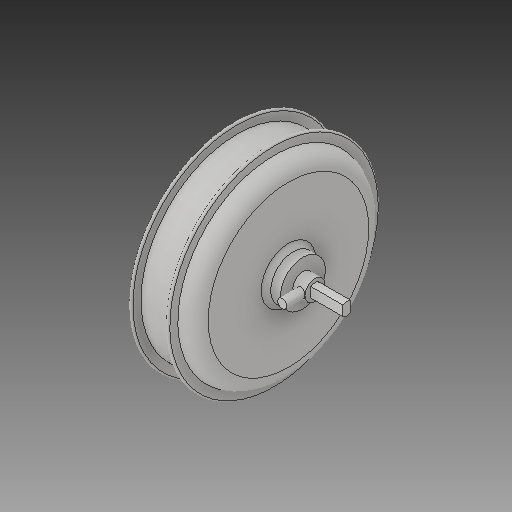
# Autodesk Inventor part: HubMotor3KW
Saved by Autodesk Inventor 2019.2 (Build 232265000, 265)
## iProperties
Created: 2018-06-05
Part Number: HubMotor3KW
Material: Generic
Document SubType Name: Modeling
Designer: eroldan
Density: 1 g/cm^3
Appearance: Default
Author: eroldan
Autodesk Inventor part; units mm, degrees
ref_plane "YZ Plane" through (0, 0, 0) normal (1, 0, 0) x (0, 1, 0)
ref_plane "XZ Plane" through (0, 0, 0) normal (0, 1, 0) x (-1, 0, 0)
ref_plane "XY Plane" through (0, 0, 0) normal (0, 0, 1) x (1, 0, 0)
sketch "Sketch1" plane through (0, 0, 0) normal (0, 0, 1) x (1, 0, 0)
  line L0 (0, 0) -> (0, 8)
  line L1 (0, 8) -> (40, 8)
  line L2 (40, 8) -> (40, 8.5)
  line L3 (40, 8.5) -> (63.75, 8.5)
  line L4 (63.75, 8.5) -> (63.75, 22.5)
  line L5 (63.75, 22.5) -> (78, 22.5)
  line L6 (78, 22.5) -> (78, 120)
  line L7 (78, 120) -> (86, 120)
  line L8 (86, 120) -> (86, 132)
  line L9 (86, 132) -> (90, 132)
  line L10 (90, 132) -> (90, 120)
  line L11 (90, 120) -> (132, 120)
  line L12 (132, 120) -> (132, 132)
  line L13 (132, 132) -> (136, 132)
  line L14 (136, 132) -> (136, 120)
  line L15 (136, 120) -> (154, 120)
  line L16 (154, 120) -> (154, 28)
  line L17 (154, 28) -> (172, 28)
  line L18 (172, 28) -> (172, 12.5)
  line L19 (172, 12.5) -> (187, 12.5)
  line L20 (187, 12.5) -> (187, 8)
  line L21 (187, 8) -> (227, 8)
  line L22 (227, 8) -> (227, 0)
  line L23 (0, 0) -> (227, 0)
  line L24 (-45.4, 0) -> (272.4, 0) projected
  point P0 (111, 120)
  point P1 (32, 8)
  dimension "d0" = 8
  dimension "d1" = 8
  dimension "d2" = 46
  dimension "d3" = 8.5
  dimension "d4" = 14.25
  dimension "d5" = 23.75
  dimension "d6" = 22.5
  dimension "d7" = 40
  dimension "d8" = 4
  dimension "d9" = 12
  dimension "d11" = 4
  dimension "d12" = 50
  dimension "d14" = 28
  dimension "d16" = 36
  dimension "d18" = 15
  dimension "d19" = 12.5
  dimension "d20" = 40
  dimension "d21" = 18
  dimension "d22" = 147
  dimension "d38" = 120
  dimension "d52" = 76
  dimension "d54" = 8
  dimension "d55" = 79
  dimension "d56" = 155
  constraints: 48 end point, 17 perpendicular, 4 horizontal alignment, 3 horizontal, 3 point on line, 3 vertical, 1 midpoint
  measures "d0" distance of L0.start L0.end
  measures "d1" distance of L6.end L7.end
  measures "d2" horizontal distance of L2.end L8.end
  measures "d3" distance from line of L0.start L3
  measures "d4" distance of L4.end L5.end
  measures "d5" distance of L2.end L3.end
  measures "d6" vertical distance of L0.start L5.end
  measures "d7" distance of L0.end L1.end
  measures "d8" distance of L8.end L9.end
  measures "d9" distance of L9.end L10.end
  measures "d11" distance of L12.end L13.end
  measures "d12" distance between parallel lines of L14 L8
  measures "d14" vertical distance of L16.end L22.end
  measures "d16" horizontal distance of L17.end L14.end
  measures "d18" distance of L18.end L19.end
  measures "d19" vertical distance of L22.end L19.end
  measures "d20" distance of L20.end L21.end
  measures "d21" distance of L14.end L15.end
  measures "d22" distance between parallel lines of L2 L20
  measures "d38" distance between parallel lines of L24 L11
  measures "d52" distance from line of L20 point (111, 120)
  measures "d54" distance of point (32, 8) L1.end
  measures "d55" horizontal distance of point (32, 8) point (111, 120)
  measures "d56" distance of point (32, 8) L20.end
revolve "Revolution1" add sketch "Sketch1" angle 360 about axis through (-10, 0, 0) along (1, 0, 0)
fillet "Fillet1" radius 20 1 edges at (154, -120, 0)
fillet "Fillet2" radius 6 1 edges at (78, -120, 0)
fillet "Fillet4" radius 2 4 edges at (132, -132, 0) (136, -132, 0) (86, -132, 0) (90, -132, 0)
fillet "Fillet6" radius 6 1 edges at (154, -28, 0)
sketch "Sketch2" plane through (0, 0, 0) normal (-1, 0, 0) x (0, 0, 1)
  line L0 (5, -10) -> (-5, -10)
  line L1 (-5, -10) -> (-5, 10)
  line L2 (-5, 10) -> (5, 10)
  line L3 (5, 10) -> (5, -10)
  line L4 (5, -10) -> (-5, 10) construction
  line L5 (-5, -10) -> (5, 10) construction
  line L6 (-13, 18) -> (-13, -18)
  line L7 (-13, -18) -> (13, -18)
  line L8 (13, -18) -> (13, 18)
  line L9 (13, 18) -> (-13, 18)
  point P0 (0, 0)
  dimension "d29" = 10
  dimension "d30" = 20
  dimension "d31" = 8
  constraints: 20 end point, 4 parallel, 2 midpoint, 2 perpendicular, 1 horizontal, 3 other
  measures "d29" distance of L1.end L2.end
  measures "d30" distance of L0.end L1.end
  measures "d31" distance from line of L2.end L8
extrude "Extrusion1" cut sketch "Sketch2" against normal up to surface (40 mm away)
sketch "Sketch3" plane through (227, 0, 0) normal (1, 0, 0) x (0, 0, -1)
  line L0 (-13, 18) -> (13, 18) projected
  line L1 (13, 18) -> (13, -18) projected
  line L2 (13, -18) -> (-13, -18) projected
  line L3 (5, 10) -> (-5, 10) projected
  line L4 (5, -10) -> (5, 10) projected
  line L5 (-5, -10) -> (5, -10) projected
  line L6 (-5, 10) -> (-5, -10) projected
  line L7 (-13, -18) -> (-13, 18) projected
  point P0 (0, 0)
extrude "Extrusion2" cut sketch "Sketch3" against normal up to surface (40 mm away)
sketch "Sketch6" plane through (40, 0, 0) normal (-1, 0, 0) x (0, 0, 1)
  circle A0 centre (0, 0) radius 12.5 projected
  arc A1 (5, 6.245) -> (-5, 6.245) centre (0, 0) ccw projected
  line L0 (-5, -6.245) -> (-5, 6.245) projected
  arc A2 (-5, -6.245) -> (5, -6.245) centre (0, 0) ccw projected
  line L1 (5, 6.245) -> (5, -6.245) projected
  arc A3 (5.7, 6.5727) -> (-5.7, 6.5727) centre (0, 0) ccw
  line L2 (5.7, 6.5727) -> (5.7, -6.5727)
  arc A4 (-5.7, -6.5727) -> (5.7, -6.5727) centre (0, 0) ccw
  line L3 (-5.7, -6.5727) -> (-5.7, 6.5727)
  dimension "d44" = 0.7
  constraints: 4 end point, 4 point on circle, 2 centre point, 3 other
  measures "d44" radial gap between concentric circles of A1 A3
extrude "Extrusion5" add sketch "Sketch6" along normal blind 4 separate body contours A0
sketch "Sketch7" plane through (36, 0, 0) normal (-1, 0, 0) x (0, 0, 1)
  line L0 (5.7, 6.5727) -> (5.7, -6.5727) projected
  arc A0 (-5.7, -6.5727) -> (5.7, -6.5727) centre (0, 0) ccw projected
  line L1 (-5.7, -6.5727) -> (-5.7, 6.5727) projected
  arc A1 (5.7, 6.5727) -> (-5.7, 6.5727) centre (0, 0) ccw projected
  circle A2 centre (0, 0) radius 12.5 projected
extrude "Extrusion6" add sketch "Sketch7" along normal blind 4 separate body
sketch "Sketch9" plane through (227, -6.245, 5) normal (0, 0, 1) x (1, 0, 0)
  line L0 (-40, -6.255) -> (-40, 18.745) construction
  circle A0 centre (-45.75, 6.245) radius 5.75
  point P0 (-227, 6.245)
  dimension "d49" = 11.5
  constraints: 1 centre point, 1 horizontal alignment, 1 tangent
  measures "d49" diameter of A0
extrude "Extrusion7" add sketch "Sketch9" along normal blind 30 bodies 1
equation "\"d11\" = d8"
body "Solid1"
body "Solid4"
body "Solid5"
